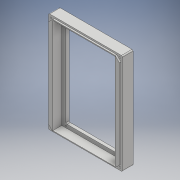
# Autodesk Inventor part: Dessus boitier
Saved by Autodesk Inventor 2018.1 (Build 221171000, 171)
## iProperties
Created: 2024-08-19
Part Number: Dessus boitier
Material: Generic
Document SubType Name: Modeling
Designer: mouta
Density: 1 g/cm^3
Appearance: Default
Author: mouta
Autodesk Inventor part; units mm, degrees
ref_plane "YZ Plane" through (0, 0, 0) normal (1, 0, 0) x (0, 1, 0)
ref_plane "XZ Plane" through (0, 0, 0) normal (0, 1, 0) x (-1, 0, 0)
ref_plane "XY Plane" through (0, 0, 0) normal (0, 0, 1) x (1, 0, 0)
sketch "Sketch1" plane through (0, 0, 0) normal (0, 1, 0) x (-1, 0, 0)
  line L0 (2, 0) -> (138, 0)
  line L1 (140, -2) -> (140, -188)
  line L2 (138, -190) -> (2, -190)
  line L3 (0, -188) -> (0, -2)
  arc A0 (140, -2) -> (138, 0) centre (138, -2) ccw
  arc A1 (2, 0) -> (0, -2) centre (2, -2) ccw
  arc A2 (0, -188) -> (2, -190) centre (2, -188) ccw
  arc A3 (138, -190) -> (140, -188) centre (138, -188) ccw
  line L4 (21, -11.5) -> (119, -11.5)
  line L5 (121, -13.5) -> (121, -176.5)
  line L6 (119, -178.5) -> (21, -178.5)
  line L7 (19, -176.5) -> (19, -13.5)
  arc A4 (121, -13.5) -> (119, -11.5) centre (119, -13.5) ccw
  arc A5 (119, -178.5) -> (121, -176.5) centre (119, -176.5) ccw
  arc A6 (19, -176.5) -> (21, -178.5) centre (21, -176.5) ccw
  arc A7 (21, -11.5) -> (19, -13.5) centre (21, -13.5) ccw
  point P0 (0, 0)
  point P1 (140, -190)
  point P2 (140, 0)
  point P3 (0, -190)
  point P4 (121, -178.5)
  point P5 (121, -11.5)
  point P6 (19, -178.5)
  dimension "d5" = 190
  dimension "d6" = 140
  dimension "d7" = 102
  dimension "d8" = 167
  dimension "d9" = 2
  dimension "d57" = 11.5
  dimension "d58" = 19
  constraints: 16 end point, 16 point on circle, 16 tangent, 14 point on line, 8 centre point, 6 equal radius, 4 parallel, 2 horizontal, 2 perpendicular
  measures "d5" distance between parallel lines of L2 L0
  measures "d6" distance between parallel lines of L3 L1
  measures "d7" distance of point (121, -178.5) point (19, -178.5)
  measures "d8" distance of point (121, -11.5) point (121, -178.5)
  measures "d9" radius of A4
  measures "d57" distance between parallel lines of L2 L6
  measures "d58" distance between parallel lines of L3 L7
extrude "Extrusion1" add sketch "Sketch1" along normal blind 20
sketch "Sketch2" plane through (0, 0, 0) normal (0, -1, 0) x (1, 0, 0)
  line L0 (-11, -3) -> (-129, -3)
  line L1 (-137, -11) -> (-137, -179)
  line L2 (-129, -187) -> (-11, -187)
  line L3 (-3, -179) -> (-3, -11)
  line L4 (-137, -179) -> (-129, -187)
  line L5 (-137, -11) -> (-129, -3)
  line L6 (-11, -3) -> (-3, -11)
  line L7 (-11, -187) -> (-3, -179)
  line L8 (-129, -187) -> (-129, -185.4)
  line L9 (-129, -185.4) -> (-11, -185.4)
  line L10 (-11, -185.4) -> (-11, -4.6)
  line L11 (-11, -4.6) -> (-129, -4.6)
  line L12 (-129, -4.6) -> (-129, -185.4)
  point P0 (0, 0)
  point P1 (-3, -3)
  point P2 (-137, -187)
  point P3 (-137, -3)
  point P4 (-3, -187)
  dimension "d86" = 134
  dimension "d87" = 184
  dimension "d88" = 8
  dimension "d89" = 8
  dimension "d90" = 8
  dimension "d91" = 8
  dimension "d92" = 8
  dimension "d93" = 8
  dimension "d94" = 8
  dimension "d95" = 8
  dimension "d96" = 1.6
  dimension "d97" = 180.8
  dimension "d98" = 180.8
  constraints: 26 end point, 9 point on line, 6 perpendicular, 2 parallel, 1 horizontal
  measures "d86" distance of point (-3, -187) point (-137, -187)
  measures "d87" distance of point (-137, -187) point (-137, -3)
  measures "d88" distance of L1.end point (-137, -187)
  measures "d89" distance of L2.start point (-137, -187)
  measures "d90" distance of L1.start point (-137, -3)
  measures "d91" distance of L0.end point (-137, -3)
  measures "d92" distance of L0.start point (-3, -3)
  measures "d93" distance of L3.end point (-3, -3)
  measures "d94" distance of L2.end point (-3, -187)
  measures "d95" distance of L3.start point (-3, -187)
  measures "d96" distance of L2.start L8.end
  measures "d97" distance of L9.end L10.end
  measures "d98" distance between parallel lines of L11 L9
extrude "Extrusion2" add sketch "Sketch2" along normal blind 3
hole "Hole1" at (-135, 20, -5) direction (0, -1, 0) diameter 3 end through all countersink diameter 5 countersink angle 90
hole "Hole2" at (-135, 20, -185) direction (0, -1, 0) diameter 3 end through all countersink diameter 5 countersink angle 90
hole "Hole3" at (-5, 20, -185) direction (0, -1, 0) diameter 3 end through all countersink diameter 5 countersink angle 90
hole "Hole4" at (-5, 20, -5) direction (0, -1, 0) diameter 3 end through all countersink diameter 5 countersink angle 90
hole "Hole5" at (-120.5, 0, -8) direction (0, 1, 0) diameter 3 depth 19 tip angle 118
hole "Hole6" at (-19.5, 0, -8) direction (0, 1, 0) diameter 3 depth 19 tip angle 118
hole "Hole7" at (-120.5, 0, -182) direction (0, 1, 0) diameter 3 depth 19 tip angle 118
hole "Hole8" at (-19.5, 0, -182) direction (0, 1, 0) diameter 3 depth 19 tip angle 118
sketch "Sketch3" plane through (0, 0, 0) normal (0, -1, 0) x (1, 0, 0)
  line L0 (-11, -185.4) -> (-11, -4.6) projected
  line L1 (-129, -4.6) -> (-11, -4.6) projected
  line L2 (-11, -185.4) -> (-129, -185.4)
  line L3 (-129, -185.4) -> (-129, -4.6)
  line L4 (-129, -4.6) -> (-11, -4.6)
  line L5 (-11, -4.6) -> (-11, -185.4)
  point P0 (0, 0)
  constraints: 8 end point, 2 parallel, 1 horizontal, 1 perpendicular
extrude "Extrusion3" cut sketch "Sketch3" against normal blind 14
equation "\"d89\" = d88"
equation "\"d90\" = d88"
equation "\"d91\" = d90"
equation "\"d92\" = d88"
equation "\"d93\" = d92"
equation "\"d94\" = d88"
equation "\"d95\" = d94"
body "Solid1"
